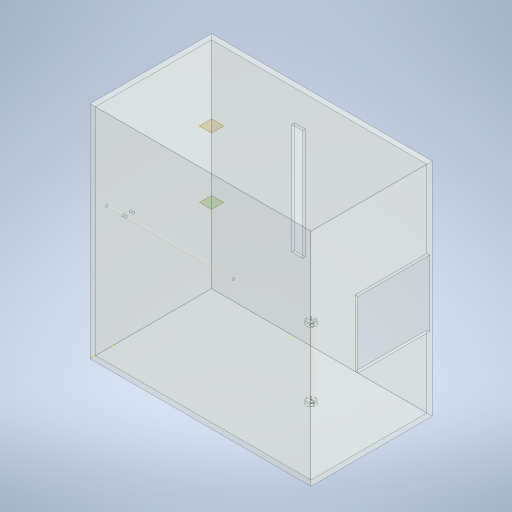
# Autodesk Inventor part: DSN 1
Saved by Autodesk Inventor 2024 (Build 280153000, 153)
## iProperties
Created: 2023-06-04
Part Number: DSN 1
Material: Glass
Document SubType Name: Modeling
Designer: hithi
Density: 2.18 g/cm^3
Appearance: Clear
Author: hithi
Autodesk Inventor part; units mm, degrees
ref_plane "YZ Plane" through (0, 0, 0) normal (1, 0, 0) x (0, 1, 0)
ref_plane "XZ Plane" through (0, 0, 0) normal (0, 1, 0) x (-1, 0, 0)
ref_plane "XY Plane" through (0, 0, 0) normal (0, 0, 1) x (1, 0, 0)
sketch "Sketch1" plane through (0, 0, 0) normal (0, 0, 1) x (1, 0, 0)
  line L0 (0, 0) -> (400, 0)
  line L1 (400, 0) -> (400, 400)
  line L2 (400, 400) -> (0, 400)
  line L3 (0, 400) -> (0, 0)
  line L4 (5, 5) -> (395, 5)
  line L5 (395, 5) -> (395, 395)
  line L6 (395, 395) -> (5, 395)
  line L7 (5, 395) -> (5, 5)
  dimension "d0" = 400
  dimension "d1" = 400
  dimension "d2" = 390
  dimension "d3" = 390
  constraints: 16 end point, 4 parallel, 2 horizontal, 2 perpendicular
  measures "d0" distance of L2.end L1.end
  measures "d1" distance of L1.end L0.end
  measures "d2" distance of L6.end L5.end
  measures "d3" distance of L5.end L4.end
extrude "Extrusion1" add sketch "Sketch1" along normal blind 170
sketch "Sketch2" plane through (0, 0, 170) normal (0, 0, 1) x (1, 0, 0)
  line L0 (400, 0) -> (400, 400) projected
  line L1 (0, 0) -> (400, 0)
  line L2 (400, 0) -> (400, 400)
  line L3 (400, 400) -> (0, 400)
  line L4 (0, 400) -> (0, 0)
  constraints: 8 end point, 2 parallel, 1 horizontal, 1 perpendicular
extrude "Extrusion2" add sketch "Sketch2" along normal blind 5
sketch "Sketch3" plane through (400, 0, 0) normal (1, 0, 0) x (0, 0, -1)
  line L0 (0, 0) -> (0, 400) projected
  line L1 (0, 140) -> (-130, 140)
  line L2 (-130, 140) -> (-130, 250)
  line L3 (-130, 250) -> (0, 250)
  line L4 (0, 250) -> (0, 140)
  dimension "d8" = 130
  dimension "d9" = 110
  constraints: 8 end point, 2 parallel, 1 horizontal, 1 perpendicular, 1 point on line
  measures "d8" distance of L2.end L3.end
  measures "d9" distance of L1.end L2.end
extrude "Extrusion3" cut sketch "Sketch3" against normal blind 5
sketch "Sketch4" plane through (400, 0, 175) normal (1, 0, 0) x (0, 0, -1)
  line L0 (45, 250) -> (45, 140) projected
  line L1 (175, 140) -> (175, 5) projected
  line L2 (45, 140) -> (175, 140)
  line L3 (175, 140) -> (175, 135)
  line L4 (175, 135) -> (45, 135)
  line L5 (45, 135) -> (45, 140)
  line L6 (175, 250) -> (45, 250) projected
  line L7 (175, 250) -> (45, 250)
  line L8 (45, 250) -> (45, 255)
  line L9 (45, 255) -> (175, 255)
  line L10 (175, 255) -> (175, 250)
  point P0 (175, 0)
  dimension "d12" = 5
  dimension "d13" = 5
  constraints: 16 end point, 4 parallel, 2 horizontal, 2 perpendicular, 2 point on line
  measures "d12" distance of L2.end L3.end
  measures "d13" distance of L7.end L8.end
extrude "Extrusion4" cut sketch "Sketch4" against normal blind 5
sketch "Sketch5" plane through (0, 0, 0) normal (0, 0, -1) x (-1, 0, 0)
  line L0 (-400, 255) -> (-400, 400) projected
  line L1 (0, 0) -> (-400, 0)
  line L2 (-400, 0) -> (-400, 400)
  line L3 (-400, 400) -> (0, 400)
  line L4 (0, 400) -> (0, 0)
  line L5 (-170, 135) -> (-150, 135)
  line L6 (-150, 135) -> (-150, 335)
  line L7 (-150, 335) -> (-170, 335)
  line L8 (-170, 335) -> (-170, 135)
  dimension "d16" = 20
  dimension "d17" = 200
  constraints: 16 end point, 4 parallel, 2 horizontal, 2 perpendicular
  measures "d16" distance of L7.end L6.end
  measures "d17" distance of L6.end L5.end
extrude "Extrusion5" add sketch "Sketch5" along normal blind 5
sketch "Sketch6" plane through (0, 0, 175) normal (-1, 0, 0) x (0, 0, 1)
  circle A0 centre (-20, 195) radius 2.5
  point P0 (-175, 0)
  dimension "d20" = 5
  constraints: 1 centre point
  measures "d20" diameter of A0
extrude "Extrusion6" cut sketch "Sketch6" against normal blind 220
sketch "Sketch7" plane through (0, 0, 175) normal (-1, 0, 0) x (0, 0, 1)
  circle A0 centre (-20, 195) radius 2.5 projected
  circle A1 centre (-20, 195) radius 2.5
  point P0 (-175, 0)
  constraints: 1 centre point, 1 coincident
extrude "Extrusion7" add sketch "Sketch7" against normal blind 200
sketch "Sketch8" plane through (0, 0, 175) normal (-1, 0, 0) x (0, 0, 1)
  circle A0 centre (-20, 195) radius 2.5 projected
  circle A1 centre (-20, 195) radius 2.5
  point P0 (-175, 0)
  constraints: 1 centre point, 1 coincident
extrude "Extrusion8" add sketch "Sketch8" along normal blind 30
sketch "Sketch9" plane through (150, 135, 0) normal (1, 0, 0) x (0, 0, -1)
  point P0 (0, -135)
sketch "Sketch10" plane through (150, 135, 0) normal (1, 0, 0) x (0, 0, -1)
  point P0 (0, -135)
sketch "Sketch11" plane through (0, 0, 175) normal (-1, 0, 0) x (0, 0, 1)
  circle A0 centre (-32.5584, 194.9375) radius 2.5
  circle A1 centre (-20, 195) radius 2.5 projected
  circle A2 centre (-20, 195) radius 2.5
  point P0 (-175, 0)
  dimension "d27" = 5
  dimension "d28" = 5
  constraints: 2 centre point, 1 coincident
  measures "d27" diameter of A0
  measures "d28" diameter of A2
extrude "Extrusion9" add sketch "Sketch11" against normal blind 200 contours A1
sketch "Sketch12" plane through (0, 0, 175) normal (-1, 0, 0) x (0, 0, 1)
  circle A0 centre (-33.2614, 194.6952) radius 2.5
  point P0 (-175, 0)
  dimension "d31" = 5
  constraints: 1 centre point
  measures "d31" diameter of A0
extrude "Extrusion10" cut sketch "Sketch12" against normal blind 200
sketch "Sketch13" plane through (0, 0, 175) normal (0, 0, 1) x (1, 0, 0)
  point P0 (0, 0)
sketch "Sketch14" plane through (0, 0, 175) normal (0, 0, 1) x (1, 0, 0)
  line L0 (400, 0) -> (0, 0) projected
  line L1 (400, 0) -> (0, 0)
  line L2 (0, 0) -> (0, 400)
  line L3 (0, 400) -> (400, 400)
  line L4 (400, 400) -> (400, 0)
  constraints: 8 end point, 2 parallel, 1 horizontal, 1 perpendicular
extrude "Extrusion11" cut sketch "Sketch14" against normal blind 5
sketch "Sketch15" plane through (0, 0, 170) normal (0, 0, 1) x (1, 0, 0)
  line L0 (0, 0) -> (0, 400) projected
  line L1 (400, 0) -> (0, 0)
  line L2 (0, 0) -> (0, 400)
  line L3 (0, 400) -> (400, 400)
  line L4 (400, 400) -> (400, 0)
  line L5 (5, 395) -> (395, 395) projected
  line L6 (395, 395) -> (395, 5) projected
  line L7 (5, 395) -> (395, 395)
  line L8 (395, 395) -> (395, 5)
  line L9 (395, 5) -> (5, 5)
  line L10 (5, 5) -> (5, 395)
  constraints: 16 end point, 4 parallel, 2 horizontal, 2 perpendicular
extrude "Extrusion12" add sketch "Sketch15" along normal blind 40
sketch "Sketch16" plane through (0, 0, 210) normal (0, 0, 1) x (1, 0, 0)
  line L0 (0, 0) -> (0, 400) projected
  line L1 (0, 400) -> (400, 400) projected
  line L2 (0, 0) -> (400, 0)
  line L3 (400, 0) -> (400, 400)
  line L4 (400, 400) -> (0, 400)
  line L5 (0, 400) -> (0, 0)
  constraints: 8 end point, 2 parallel, 1 horizontal, 1 perpendicular
extrude "Extrusion13" add sketch "Sketch16" along normal blind 5
ref_plane "Work Plane3" through (0, 135, -5) normal (0, -1, 0) x (1, 0, 0)
sketch "Sketch17" plane through (0, 135, -5) normal (0, -1, 0) x (1, 0, 0)
  line L0 (0, 220) -> (400, 220) projected
  circle A0 centre (400, 220) radius 8.2953
  circle A1 centre (402.9982, 221.2832) radius 3.0106
  point P0 (0, 5)
  constraints: 2 centre point
extrude "Extrusion14" add sketch "Sketch17" along normal blind 5
ref_plane "Work Plane4" through (0, 255, -5) normal (0, 1, 0) x (1, 0, 0)
sketch "Sketch18" plane through (0, 255, -5) normal (0, 1, 0) x (1, 0, 0)
  line L0 (400, -220) -> (400, 0) projected
  circle A0 centre (400, -220) radius 8.3192
  circle A1 centre (403.115, -221.3029) radius 3.1274
  point P0 (0, -5)
  constraints: 2 centre point
extrude "Extrusion15" add sketch "Sketch18" along normal blind 5
sketch "Sketch19" plane through (0, 0, 215) normal (0, 0, 1) x (1, 0, 0)
  line L0 (400, 400) -> (0, 400) projected
  line L1 (0, 0) -> (400, 0)
  line L2 (400, 0) -> (400, 400)
  line L3 (400, 400) -> (0, 400)
  line L4 (0, 400) -> (0, 0)
  constraints: 8 end point, 2 parallel, 1 horizontal, 1 perpendicular
extrude "Extrusion16" cut sketch "Sketch19" against normal blind 5
sketch "Sketch20" plane through (0, 130, -5) normal (0, -1, 0) x (1, 0, 0)
  circle A0 centre (403.1559, 221.2408) radius 2.8533
  point P0 (0, 5)
  constraints: 1 centre point
extrude "Extrusion17" cut sketch "Sketch20" against normal blind 130
sketch "Sketch21" plane through (0, 255, -5) normal (0, -1, 0) x (1, 0, 0)
  circle A0 centre (403.1087, 221.3826) radius 2.5
  point P0 (0, 5)
  dimension "d50" = 5
  constraints: 1 centre point
  measures "d50" diameter of A0
extrude "Extrusion18" add sketch "Sketch21" along normal blind 120
sketch "Sketch22" plane through (0, 0, 210) normal (0, 0, 1) x (1, 0, 0)
  point P0 (0, 0)
sketch "Sketch23" plane through (0, 0, 210) normal (0, 0, 1) x (1, 0, 0)
  line L0 (0, 0) -> (0, 400) projected
  line L1 (400, 400) -> (400, 260) projected
  line L2 (0, 0) -> (400, 0)
  line L3 (400, 0) -> (400, 400)
  line L4 (400, 400) -> (0, 400)
  line L5 (0, 400) -> (0, 0)
  constraints: 8 end point, 2 parallel, 1 horizontal, 1 perpendicular
extrude "Extrusion19" add sketch "Sketch23" along normal blind 5
body "Solid1"
